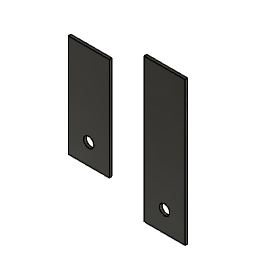
Top anvil mounts (Autodesk Fusion 360 design; units mm, degrees)
Autodesk Fusion 360 part; units mm, degrees
sketch "Sketch1" plane through (0, 0, 0) normal (0, 1, 0) x (1, 0, 0)
  line L0 (-38.1, 50.8) -> (-88.9, 50.8)
  line L1 (-88.9, 50.8) -> (-88.9, -76.2)
  line L2 (-88.9, -76.2) -> (-38.1, -76.2)
  line L3 (-38.1, -76.2) -> (-38.1, 50.8)
  line L4 (55.88, 76.2) -> (5.08, 76.2)
  line L5 (5.08, 76.2) -> (5.08, -101.6)
  line L6 (5.08, -101.6) -> (55.88, -101.6)
  line L7 (55.88, -101.6) -> (55.88, 76.2)
  line L8 (-63.5, 50.8) -> (-63.5, 25.4) construction
  line L9 (30.48, 76.2) -> (30.48, 50.8) construction
  circle A0 centre (-63.5, 25.4) radius 6.35
  circle A1 centre (30.48, 50.8) radius 6.35
  point P0 (-63.5, 0)
  point P1 (30.48, 0)
  dimension "d1" = 50.8
  dimension "d2" = 127
  dimension "d3" = 50.8
  dimension "d4" = 177.8
  constraint horizontal L0
  constraint perpendicular L0 L1
  constraint parallel L0 L2
  constraint parallel L1 L3
  constraint horizontal L4
  constraint perpendicular L4 L5
  constraint parallel L4 L6
  constraint parallel L5 L7
  constraint midpoint L0 L8.start
  constraint perpendicular L0 L8
  constraint midpoint L4 L9.start
  constraint perpendicular L4 L9
  constraint coincident L8.end A0.centre
  constraint coincident L9.end A1.centre
  measures "d1" distance of L1.end L2.end
  measures "d2" distance of L0.end L1.end
  measures "d3" distance of L5.end L6.end
  measures "d4" distance of L4.end L5.end
extrude "Extrude1" add sketch "Sketch1" along normal blind 3.175 makes body 1 at (-63.3418, 0, 44.4441) makes body 2 at (30.6382, 0, 52.9107)
copy_body "Body->Comp1" bodies 1 removing the originals makes body 3 in component "Small Top Anvil Mount"
copy_body "Body->Comp2" bodies 2 removing the originals makes body 4 in component "Tall Top Anvil Mount"
component "Small Top Anvil Mount" placed x (1, 0, 0) y (0, 1, 0) z (0, 0, 1) at (0, 0, 0)
component "Tall Top Anvil Mount" placed x (1, 0, 0) y (0, 1, 0) z (0, 0, 1) at (0, 0, 0)
equation "d9 = ( 1 / 8 ) * 1 in"
named bodies: "Small Top Anvil Mount", "Tall Top Anvil Mount"
